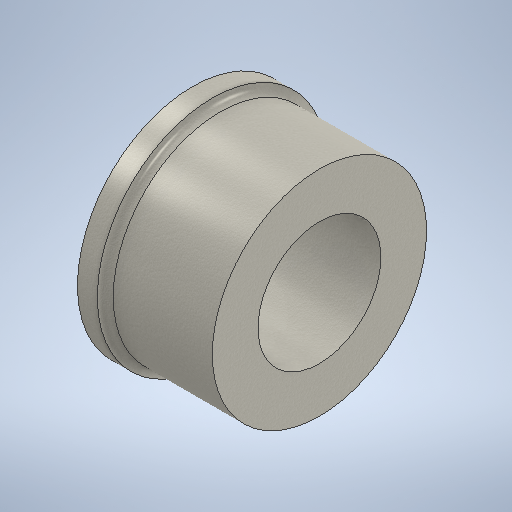
# Autodesk Inventor part: Laufrad
Saved by Autodesk Inventor 2025.2 (Build 292293000, 293)
## iProperties
Created: 2025-02-03
Part Number: Laufrad
Material: Generisch
Document SubType Name: Modeling
Designer: unter
Density: 1 g/cm^3
Appearance: Vorgabe
Author: unter
Autodesk Inventor part; units mm, degrees
ref_plane "YZ Plane" through (0, 0, 0) normal (1, 0, 0) x (0, 1, 0)
ref_plane "XZ Plane" through (0, 0, 0) normal (0, 1, 0) x (-1, 0, 0)
ref_plane "XY Plane" through (0, 0, 0) normal (0, 0, 1) x (1, 0, 0)
derived "Skelett_Laufkatze.ipt"
sketch "Laufrad" plane through (-97, 65, 62.4) normal (0, 0, -1) x (-1, 0, 0)
  line L0 (34, 50) -> (0, 50) construction
  line L1 (34, 50) -> (34, 0) construction
  line L2 (34, 40) -> (34, 10) construction
  line L3 (34, 25) -> (32, 25) construction
  line L4 (32, 25) -> (17, 25) construction
  line L5 (17, 25) -> (-47, 25)
  line L6 (17, 50) -> (17, 83)
  line L7 (17, 83) -> (7, 83)
  line L8 (3, 79) -> (-47, 79)
  line L9 (-47, 79) -> (-47, 56)
  line L10 (-47, 56) -> (0, 56)
  line L11 (0, 56) -> (0, 50)
  line L12 (0, 50) -> (17, 50)
  arc A0 (3, 79) -> (7, 83) centre (3, 83) ccw
  point P0 (-97, -65)
revolve "Umdrehung1" add sketch "Laufrad" angle 360 about axis through (-114, 90, 62.4) along (1, 0, 0)
